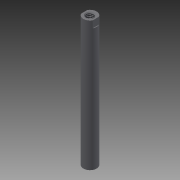
# Autodesk Inventor part: 022.452.45-FO1_BM_rod
Saved by Autodesk Inventor 2014 (Build 180170000, 170)
## iProperties
Category: PARTsolutions
Company: BIMBA
Created: 2014-01-19
Part Number: 022.452.45-FO1_BM_rod
Material: Generic
Catalog Web Link: www.cadenas.de
Description: FO1_basic_model_rod-Bimba FLAT-1
Vendor: BIMBA
Document SubType Name: Standard Catalog Part
Designer: Andrew Toennies
Manufacturer: BIMBA
Density: 1 g/cm^3
Appearance: RGB(180.00000447034725,180.00000447034725,180.00000447034725)
PSOL_IDENT_0: {$CADENAS_DATA\23d-libs\bimba\bimba\bimba_imperial\bimba_full_line\flat_cylinders\fo1\fo1_basic_mode
PSOL_IDENT_1: l_rod.prj},219 {VTYP=3D},{NB=022.452.45-FO1_BM_rod},{LINA=022.452.45-FO1_BM_rod},{NN=FO1_basic_model
PSOL_IDENT_2: _rod},{DATE=19.11.2012 05:49:13},{GEOMDATE=18.07.2011 10:15:00},{VERSION=},{LINEID=10},{LINESUBID=-1
PSOL_IDENT_3: },{WBVAR=STROKE,LENGTH,ER,RT,HR}  {NB=022.452.45-FO1_BM_rod},{LINA=022.452.45-FO1_BM_rod},{KT=DUMMY}
PSOL_IDENT_4: ,{PN=022.452.45-FO1_BM_rod},{BORE=0.56250000},{BOREPN=02},{STROKE=2.45},{STROKEMIN=0.46},{LENGTHALG=
PSOL_IDENT_5: 2.45},{LENGTH=2.45},{ER=},{RT=},{HR=},{HRALG='','N/A'},{EE=},{EEALG='','Without Extra Extension','EE'
PSOL_IDENT_6: ,'With Extra Extension'},{EELALG=0},{EELMAX=17.55},{EEL=0},{EELPN=},{A=1.12000000},{BA=0.56000},{BB=
PSOL_IDENT_7: 0.69000},{BC=1.96},{BD=2.14},{C=0.88000000},{DD=2.00000000},{D=0.11200000},{CPIL=0.12000000},{DC=0.1
PSOL_IDENT_8: 8800000},{DCP=0.12000000},{DCD=0.85500000},{ES=0.16400000},{EC=0.16400000},{ED=0.46000000},{F=0.2500
PSOL_IDENT_9: 0000},{H=0.22000000},{J=0.34000000},{K=0.14000000},{L=0.19000000},{LDP=0.20000000},{LP=0.16000000},{
PSOL_IDENT_10: LPDP=0.28000000},{TD=0.65700000},{TDDP=0.10000},{TD1=0.59500},{TD2=0.61000},{TDIN=0.56200},{LSF=0.31
PSOL_IDENT_11: 250000},{LSFDP=0.02000000},{BC1=0.81000},{BC2=1.38000},{BC3=1.96000},{BC4=2.52000},{BD1=1.06000},{BD
PSOL_IDENT_12: 2=1.62000},{BD3=2.14000},{BD4=2.70000},{MT=0.16400000},{CMT=0.16400000},{LG=0.38000000},{HF=0.140000
PSOL_IDENT_13: 00},{HM=0.00000000},{HD=0.14},{HALG=0},{HDY=0.46},{HDH=1.53},{LG1=0.00000000}
CNS_NN: FO1_basic_model_rod
CNS_NT: Bimba FLAT-1
CNS_NB: 022.452.45-FO1_BM_rod
CNS_NBSYN: $PN.
CNS_LINA: 022.452.45-FO1_BM_rod
CNS_PN: 022.452.45-FO1_BM_rod
CNS_BORE: 9/16
CNS_BOREPN: 02
CNS_STROKE: 2.45
CNS_STROKEMIN: 0.460
CNS_LENGTHALG: 2.450
CNS_LENGTH: 2.45
CNS_ER: Single End Rod
CNS_RT: Standard
CNS_HR: N/A
CNS_HRALG: '','N/A'
CNS_EEALG: '','Without Extra Extension','EE','With Extra Extension'
CNS_EELALG: 0
CNS_EELMAX: 17.550
CNS_EEL: 0.000
CNS_A: 1.12000000
CNS_BA: 0.56000
CNS_BB: 0.69000
CNS_BC: 1.960
CNS_BD: 2.140
CNS_C: 0.88000000
CNS_DD: 2.00000000
CNS_D: 0.11200000
CNS_CPIL: 0.12000000
CNS_DC: 0.18800000
CNS_DCP: 0.12000000
CNS_DCD: 0.85500000
CNS_ES: 0.16400000
CNS_EC: 0.16400000
CNS_ED: 0.46000000
CNS_F: 0.25000000
CNS_H: 0.22000000
CNS_J: 0.34000000
CNS_K: 0.14000000
CNS_L: 0.19000000
CNS_LDP: 0.20000000
CNS_LP: 0.16000000
CNS_LPDP: 0.28000000
CNS_TD: 0.65700000
CNS_TDDP: 0.10000
CNS_TD1: 0.59500
CNS_TD2: 0.61000
CNS_TDIN: 0.56200
CNS_LSF: 0.31250000
CNS_LSFDP: 0.02000000
CNS_BC1: 0.81000
CNS_BC2: 1.38000
CNS_BC3: 1.96000
CNS_BC4: 2.52000
CNS_BD1: 1.06000
CNS_BD2: 1.62000
CNS_BD3: 2.14000
CNS_BD4: 2.70000
CNS_MT: 0.16400000
CNS_CMT: 0.16400000
CNS_LG: 0.38000000
CNS_HF: 0.14000000
CNS_HM: 0.00000000
CNS_HD: 0.140
CNS_HALG: 0.000
CNS_HDY: 0.460
CNS_HDH: 1.530
CNS_LG1: 0.00000000
SUPPLIER: BIMBA
ARTICLENO: 022.452.45-FO1_BM_rod
BOMINFO: 022.452.45-FO1_BM_rod
CREATOR: CADENAS GmbH
Title: 022.452.45-FO1_BM_rod
Author: Cadenas PARTsolutions
Comments: Bimba FLAT-1
Autodesk Inventor part; units mm, degrees
ref_plane "YZ Plane" through (0, 0, 0) normal (1, 0, 0) x (0, 1, 0)
ref_plane "XZ Plane" through (0, 0, 0) normal (0, 1, 0) x (-1, 0, 0)
ref_plane "XY Plane" through (0, 0, 0) normal (0, 0, 1) x (1, 0, 0)
sketch "Sketch_1" plane through (0, 0, 0) normal (0, 0, 1) x (1, 0, 0)
  line L0 (0, 0) -> (0, 62.23)
  line L1 (0, 62.23) -> (3.175, 62.23)
  line L2 (3.175, 62.23) -> (3.175, 0)
  line L3 (3.175, 0) -> (0, 0)
  line L4 (0, 0) -> (0, 62.23)
  constraints: 10 end point
revolve "Revolution1" add sketch "Sketch_1" angle 360 about axis through (0, 0, 0) along (0, -1, 0)
sketch "Sketch2" plane through (0, 62.23, 0) normal (0, 1, 0) x (1, 0, 0)
  point P0 (0, 0)
hole "Hole1" at (0, 62.23, 0) direction (0, -1, 0) diameter 3.4036 depth 11.684 countersink diameter 4.1656 countersink angle 90 thread size "8-36 UNF" class "2B" standard "ANSI Unified Screw Threads"
sketch "Sketch_29" plane through (0, 62.23, 0) normal (0, 1, 0) x (1, 0, 0)
  line L0 (-5.588, 12.7) -> (-5.588, -12.7)
  line L1 (-5.588, -12.7) -> (5.588, -12.7)
  line L2 (5.588, -12.7) -> (5.588, 12.7)
  line L3 (5.588, 12.7) -> (-5.588, 12.7)
  line L4 (-2.794, 6.35) -> (-2.794, -6.35)
  line L5 (-2.794, -6.35) -> (2.794, -6.35)
  line L6 (2.794, -6.35) -> (2.794, 6.35)
  line L7 (2.794, 6.35) -> (-2.794, 6.35)
  constraints: 16 end point
extrude "Extrusion1" cut sketch "Sketch_29" against normal blind 3.302
ref_plane "b11_XY" through (0, 0, 0) normal (0, 1, 0) x (1, 0, 0)
ref_plane "b11_YZ" through (0, 0, 0) normal (1, 0, 0) x (0, 0, -1)
ref_plane "b11_ZX" through (0, 0, 0) normal (0, 0, -1) x (0, 1, 0)
ref_plane "b2_XY" through (0, 62.23, 0) normal (0, 1, 0) x (1, 0, 0)
ref_plane "b2_YZ" through (0, 62.23, 0) normal (1, 0, 0) x (0, 0, -1)
ref_plane "b2_ZX" through (0, 62.23, 0) normal (0, 0, -1) x (0, 1, 0)
ref_plane "e1_XY" through (0, 62.23, -2.0828) normal (1, 0, 0) x (0, 0, -1)
ref_plane "e1_YZ" through (0, 62.23, -2.0828) normal (0, 0, -1) x (0, 1, 0)
ref_plane "e1_ZX" through (0, 62.23, -2.0828) normal (0, 1, 0) x (1, 0, 0)
ref_plane "e2_XY" through (0, 62.23, 2.0828) normal (1, 0, 0) x (0, 0, -1)
ref_plane "e2_YZ" through (0, 62.23, 2.0828) normal (0, 0, -1) x (0, 1, 0)
ref_plane "e2_ZX" through (0, 62.23, 2.0828) normal (0, 1, 0) x (1, 0, 0)
ref_plane "f1_XY" through (0, 62.23, 3.175) normal (1, 0, 0) x (0, 0, -1)
ref_plane "f1_YZ" through (0, 62.23, 3.175) normal (0, 0, -1) x (0, 1, 0)
ref_plane "f1_ZX" through (0, 62.23, 3.175) normal (0, 1, 0) x (1, 0, 0)
ref_plane "f2_XY" through (0, 62.23, -3.175) normal (1, 0, 0) x (0, 0, -1)
ref_plane "f2_YZ" through (0, 62.23, -3.175) normal (0, 0, -1) x (0, 1, 0)
ref_plane "f2_ZX" through (0, 62.23, -3.175) normal (0, 1, 0) x (1, 0, 0)
ref_plane "h1_XY" through (-2.794, 62.23, 0) normal (0, 1, 0) x (1, 0, 0)
ref_plane "h1_YZ" through (-2.794, 62.23, 0) normal (1, 0, 0) x (0, 0, -1)
ref_plane "h1_ZX" through (-2.794, 62.23, 0) normal (0, 0, -1) x (0, 1, 0)
ref_plane "h2_XY" through (2.794, 62.23, 0) normal (0, 1, 0) x (1, 0, 0)
ref_plane "h2_YZ" through (2.794, 62.23, 0) normal (1, 0, 0) x (0, 0, -1)
ref_plane "h2_ZX" through (2.794, 62.23, 0) normal (0, 0, -1) x (0, 1, 0)
ref_plane "rod_XY" through (0, 62.23, 0) normal (0, 1, 0) x (1, 0, 0)
ref_plane "rod_YZ" through (0, 62.23, 0) normal (1, 0, 0) x (0, 0, -1)
ref_plane "rod_ZX" through (0, 62.23, 0) normal (0, 0, -1) x (0, 1, 0)
ref_plane "rod_to_part_XY" through (0, 0, 0) normal (0, 1, 0) x (1, 0, 0)
ref_plane "rod_to_part_YZ" through (0, 0, 0) normal (1, 0, 0) x (0, 0, -1)
ref_plane "rod_to_part_ZX" through (0, 0, 0) normal (0, 0, -1) x (0, 1, 0)
ref_plane "to_rod_pivot_XY" through (0, 62.23, 0) normal (0, 1, 0) x (1, 0, 0)
ref_plane "to_rod_pivot_YZ" through (0, 62.23, 0) normal (1, 0, 0) x (0, 0, -1)
ref_plane "to_rod_pivot_ZX" through (0, 62.23, 0) normal (0, 0, -1) x (0, 1, 0)
ref_plane "to_rod_pivot1_XY" through (0, 0, 0) normal (0, 1, 0) x (1, 0, 0)
ref_plane "to_rod_pivot1_YZ" through (0, 0, 0) normal (1, 0, 0) x (0, 0, -1)
ref_plane "to_rod_pivot1_ZX" through (0, 0, 0) normal (0, 0, -1) x (0, 1, 0)
body "Solid1"
